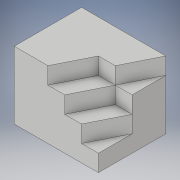
# Autodesk Inventor part: 零件23
Saved by Autodesk Inventor 2019 (Build 230136000, 136)
## iProperties
Created: 2020-09-18
Part Number: 零件23
Material: 一般
Document SubType Name: Modeling
Designer: jay
Density: 1 g/cm^3
Appearance: 預設
Author: jay
Autodesk Inventor part; units mm, degrees
ref_plane "YZ Plane" through (0, 0, 0) normal (1, 0, 0) x (0, 1, 0)
ref_plane "XZ Plane" through (0, 0, 0) normal (0, 1, 0) x (-1, 0, 0)
ref_plane "XY Plane" through (0, 0, 0) normal (0, 0, 1) x (1, 0, 0)
sketch "草圖1" plane through (0, 0, 0) normal (0, 0, 1) x (1, 0, 0)
  line L0 (0, 0) -> (50, 0)
  line L1 (50, 0) -> (50, 40)
  line L2 (50, 40) -> (0, 40)
  line L3 (0, 40) -> (0, 0)
  dimension "d0" = 50
  dimension "d1" = 40
  constraints: 8 end point, 2 parallel, 1 horizontal, 1 perpendicular
  measures "d0" distance of L1.end L2.end
  measures "d1" distance of L0.end L1.end
extrude "擠出1" add sketch "草圖1" along normal blind 40
sketch "草圖2" plane through (0, 40, 0) normal (0, 1, 0) x (1, 0, 0)
  line L0 (50, 0) -> (0, 0) projected
  line L1 (0, 0) -> (0, -40) projected
  line L2 (50, -40) -> (0, -40) construction
  line L3 (50, 0) -> (50, -40) construction
  line L4 (0, -40) -> (50, -40) projected
  line L5 (20, -40) -> (30, -20)
  line L6 (30, -20) -> (40, -20)
  line L7 (40, -20) -> (30, -40)
  line L8 (50, 0) -> (50, -40) projected
  line L9 (40, -20) -> (50, 0)
  line L10 (50, 0) -> (50, -20)
  line L11 (40, -20) -> (50, -20)
  line L12 (30, -40) -> (20, -40)
  point P0 (0, 0)
  dimension "d4" = 20
  dimension "d5" = 10
  dimension "d6" = 20
  dimension "d7" = 10
  constraints: 14 end point, 2 parallel, 2 point on line, 1 midpoint
  measures "d4" distance from line of L3 L7.end
  measures "d5" distance from line of L3 L6.end
  measures "d6" distance between parallel lines of L2 L6
  measures "d7" distance of L7.end L5.start
extrude "擠出2" cut sketch "草圖2" against normal blind 10 contours L8 L11 L9 | L7 L4 L5 L6
sketch "草圖3" plane through (30, 40, 40) normal (0, 1, 0) x (1, 0, 0)
  line L0 (20, 20) -> (10, 20) projected
  line L1 (10, 20) -> (0, 0) projected
  line L2 (20, 0) -> (0, 0) projected
  line L3 (20, 20) -> (20, 0) projected
  point P0 (-30, 40)
extrude "擠出3" cut sketch "草圖3" against normal blind 20
sketch "草圖4" plane through (30, 20, 40) normal (0, 1, 0) x (1, 0, 0)
  line L0 (10, 20) -> (20, 20) projected
  line L1 (0, 0) -> (10, 20) projected
  line L2 (20, 0) -> (0, 0) projected
  line L3 (20, 20) -> (20, 0) projected
  line L4 (20, 20) -> (10, 0)
  line L5 (10, 20) -> (0, 0) projected
  point P0 (-30, 40)
  constraints: 2 end point, 1 midpoint, 1 parallel
extrude "擠出4" cut sketch "草圖4" against normal blind 10 contours L3 L2 L4
